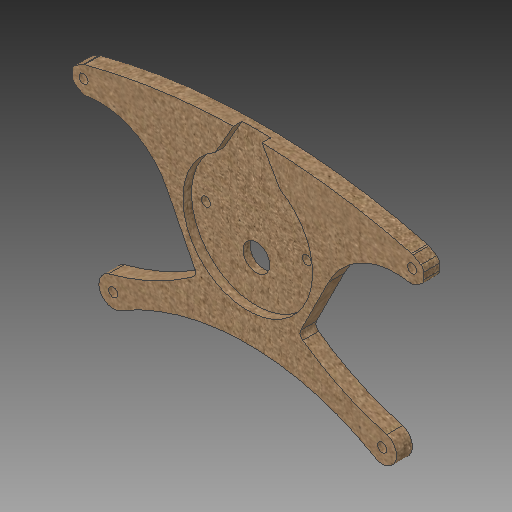
# Autodesk Inventor part: ステッピング固定具
Saved by Autodesk Inventor 2018 (Build 220112000, 112)
## iProperties
Created: 2018-08-16
Part Number: ステッピング固定具
Material: MDF 中密度繊維ボード
Document SubType Name: Modeling
Designer: shun2
Density: 0.8 g/cm^3
Appearance: ダンボール - 段ボール紙
Author: shun2
Autodesk Inventor part; units mm, degrees
ref_plane "YZ Plane" through (0, 0, 0) normal (1, 0, 0) x (0, 1, 0)
ref_plane "XZ Plane" through (0, 0, 0) normal (0, 1, 0) x (-1, 0, 0)
ref_plane "XY Plane" through (0, 0, 0) normal (0, 0, 1) x (1, 0, 0)
sketch "スケッチ1" plane through (0, 0, 0) normal (0, 0, 1) x (1, 0, 0)
  circle A0 centre (19.2131, 26.9091) radius 1.6
  circle A1 centre (8.9167, 85.9091) radius 1.6
  circle A2 centre (122.9167, 85.9091) radius 1.6
  circle A3 centre (112.6203, 26.909) radius 1.6
  line L0 (65.9168, 92.271) -> (65.9166, 46.271)
  line L1 (7.2067, 85.9091) -> (10.6267, 85.9091)
  line L2 (8.9167, 84.1991) -> (8.9167, 87.6191)
  line L3 (124.6267, 85.9091) -> (121.2067, 85.9091)
  line L4 (122.9167, 84.1991) -> (122.9167, 87.6191)
  line L5 (6.0567, 82.7816) -> (8.3869, 81.4363)
  line L6 (5.0567, 86.8043) -> (5.0567, 84.5137)
  line L7 (123.7023, 81.4412) -> (126.0241, 82.7816)
  circle A4 centre (65.9167, 59.1833) radius 4.65
  circle A5 centre (65.9167, 67.1833) radius 14
  line L8 (82.734, 67.2168) -> (82.7592, 67.2168)
  circle A6 centre (48.4167, 67.2168) radius 1.6
  circle A7 centre (83.4167, 67.2168) radius 1.6
  arc A8 (37.9167, 67.2167) -> (9.7534, 81.2022) centre (14.5444, 55.5004) ccw
  arc A9 (122.3194, 81.2102) -> (93.9167, 67.2168) centre (117.3134, 55.5494) ccw
  line L9 (37.9167, 67.2167) -> (47.5918, 47.9164)
  line L10 (93.9167, 67.2168) -> (84.2485, 47.9303)
  arc A10 (46.8453, 45.3126) -> (47.5918, 47.9164) centre (45.8039, 47.0201) ccw
  arc A11 (84.2485, 47.9303) -> (85.0094, 45.3179) centre (86.0364, 47.034) ccw
  circle A12 centre (19.2131, 26.9091) radius 1.6
  circle A13 centre (112.6203, 26.909) radius 1.6
  circle A14 centre (122.9167, 85.9091) radius 1.6
  circle A15 centre (8.9167, 85.9091) radius 1.6
  arc A16 (122.7823, 90.3275) -> (9.2985, 90.3275) centre (66.0404, -124.0864) ccw
  arc A17 (123.2706, 90.1261) -> (122.7823, 90.3275) centre (122.2706, 88.394) ccw
  arc A18 (126.0241, 82.7816) -> (127.0241, 84.5137) centre (125.0241, 84.5137) ccw
  arc A19 (122.3194, 81.2102) -> (123.7023, 81.4412) centre (122.7023, 83.1732) ccw
  arc A20 (9.2985, 90.3275) -> (8.8102, 90.1261) centre (9.8102, 88.394) ccw
  arc A21 (8.3869, 81.4363) -> (9.7534, 81.2022) centre (9.3869, 83.1683) ccw
  arc A22 (6.0567, 88.5363) -> (5.0567, 86.8043) centre (7.0567, 86.8043) ccw
  arc A23 (5.0567, 84.5137) -> (6.0567, 82.7816) centre (7.0567, 84.5137) ccw
  line L11 (8.8102, 90.1261) -> (6.0567, 88.5363)
  line L12 (123.2706, 90.1261) -> (126.0241, 88.5363)
  line L13 (127.0241, 84.5137) -> (127.0241, 86.8043)
  arc A24 (127.0241, 86.8043) -> (126.0241, 88.5363) centre (125.0241, 86.8043) ccw
  arc A25 (14.749, 29.1208) -> (22.1634, 22.8946) centre (19.2131, 26.9091) ccw
  arc A26 (109.6696, 22.8946) -> (117.0846, 29.1208) centre (112.6203, 26.909) ccw
  arc A27 (109.6696, 22.8946) -> (22.1634, 22.8946) centre (65.9165, -52.1885) ccw
  arc A28 (18.2456, 31.7962) -> (22.1634, 22.8946) centre (19.2131, 26.9091) ccw
  arc A29 (109.6696, 22.8946) -> (113.5922, 31.7955) centre (112.6203, 26.909) ccw
  arc A30 (17.6131, 31.6271) -> (46.8453, 45.3126) centre (-5.3123, 118.6583) ccw
  arc A31 (85.0094, 45.3179) -> (114.2208, 31.6271) centre (137.191, 118.6465) ccw
  point P0 (0, 0)
  dimension "d10" = 28
  dimension "d13" = 17.5
  dimension "d15" = 17.5
  dimension "d20" = 3.2
  dimension "d27" = 2.681
  dimension "d28" = 2.2906
  dimension "d29" = 2
  dimension "d31" = 2.2906
  dimension "d35" = 46.7037
  dimension "d36" = 46.7035
  dimension "d39" = 90
  dimension "d40" = 90
  constraints: 44 point on circle, 32 centre point, 28 end point, 12 tangent, 8 coincident, 3 equal radius, 1 horizontal, 1 point on line, 1 vertical
  measures "d10" distance of L10.start A5.centre
  measures "d13" distance of A6.centre A5.centre
  measures "d15" distance of A7.centre A5.centre
  measures "d20" diameter of A15
  measures "d27" distance of L7.start L7.end
  measures "d28" distance of L13.start L13.end
  measures "d29" radius of A19
  measures "d31" distance of L6.start L6.end
  measures "d35" distance from line of A3.centre L0
  measures "d36" horizontal distance of A0.centre L0.end
  measures "d39" radius of A30
  measures "d40" radius of A31
extrude "押し出し1" add sketch "スケッチ1" along normal blind 5.5 contours A5 L0 A4 | L0 A4 A5 | A23 L6 A22 L11 A20 A16 A17 L12 A24 L13 A18 L7 A19 A9 L10 A11 A31 A29 A26 A27 A25 A28 A30 A10 L9 A8 A21 L5
sketch "スケッチ3" plane through (0, 0, 5.5) normal (0, 0, 1) x (1, 0, 0)
  circle A0 centre (48.4167, 67.2168) radius 1.6 projected
  circle A1 centre (83.4167, 67.2168) radius 1.6 projected
  arc A2 (54.6667, 86.7024) -> (77.1667, 86.7024) centre (65.9167, 67.2168) ccw
  line L0 (54.6667, 86.7024) -> (60.9878, 97.6509)
  arc A3 (122.7823, 90.3275) -> (9.2985, 90.3275) centre (66.0404, -124.0864) ccw projected
  line L1 (77.1667, 86.7024) -> (70.8424, 97.6564)
  arc A4 (70.8424, 97.6564) -> (60.9878, 97.6509) centre (66.0404, -124.0864) ccw
  line L2 (60.9878, 97.6509) -> (54.6667, 86.7024)
  arc A5 (70.8424, 97.6564) -> (60.9878, 97.6509) centre (66.0404, -124.0864) ccw
  line L3 (70.8424, 97.6564) -> (77.1667, 86.7024)
  point P0 (0, 0)
  constraints: 8 end point, 8 point on circle, 3 centre point, 2 collinear, 1 concentric
extrude "押し出し2" cut sketch "スケッチ3" against normal blind 3
